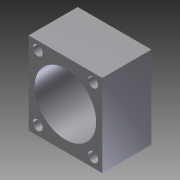
# Autodesk Inventor part: glass socket
Saved by Autodesk Inventor 2011 (Build 150239000, 239)
## iProperties
Created: 2013-10-30
Part Number: glass socket
Document SubType Name: Modeling
Designer: Devon
Density: 1 g/cm^3
Author: Devon
Autodesk Inventor part; units mm, degrees
ref_plane "YZ Plane" through (0, 0, 0) normal (1, 0, 0) x (0, 1, 0)
ref_plane "XZ Plane" through (0, 0, 0) normal (0, 1, 0) x (-1, 0, 0)
ref_plane "XY Plane" through (0, 0, 0) normal (0, 0, 1) x (1, 0, 0)
sketch "Sketch1" plane through (0, 0, 0) normal (0, 0, 1) x (1, 0, 0)
  line L0 (-26.7465, 47.6774) -> (49.4535, 47.6774)
  line L1 (49.4535, 47.6774) -> (49.4535, -37.4126)
  line L2 (49.4535, -37.4126) -> (-26.7465, -37.4126)
  line L3 (-26.7465, -37.4126) -> (-26.7465, 47.6774)
  line L4 (-26.7465, 47.6774) -> (-9.2459, 47.6774)
  line L5 (49.4535, 47.6774) -> (31.9529, 47.6774)
  line L6 (49.4535, 47.6774) -> (49.4535, 41.683)
  line L7 (49.4535, -37.4126) -> (49.4535, -31.4182)
  circle A0 centre (11.3535, 5.1324) radius 31.75
  line L8 (-26.7465, 47.6774) -> (-17.2215, 47.6774)
  line L9 (49.4535, 47.6774) -> (39.9285, 47.6774)
  line L10 (-26.7465, -37.4126) -> (-26.7465, -27.8876)
  circle A1 centre (-17.2215, -27.8876) radius 2.7813
  circle A2 centre (39.9285, -27.8876) radius 2.7813
  circle A3 centre (39.9285, 38.9906) radius 2.7813
  line L11 (-26.7465, -27.8876) -> (-17.2215, -27.8876)
  circle A4 centre (-17.2215, 38.9906) radius 2.7813
  point P0 (0, 0)
  dimension "d0" = 76.2
  dimension "d1" = 85.09
  dimension "d2" = 17.5006
  dimension "d3" = 17.5006
  dimension "d4" = 5.9944
  dimension "d5" = 5.9944
  dimension "d25" = 63.5
  dimension "d26" = 9.525
  dimension "d30" = 9.525
  dimension "d31" = 5.5626
  dimension "d32" = 5.5626
  dimension "d45" = 5.5626
  dimension "d46" = 9.525
  dimension "d48" = 5.5626
  constraints: 24 end point, 7 point on line, 5 centre point, 2 parallel, 1 coincident, 1 horizontal, 1 perpendicular
  measures "d0" distance of L1.end L2.end
  measures "d1" distance of L0.end L1.end
  measures "d2" distance of L0.start L4.end
  measures "d3" distance of L0.end L5.end
  measures "d4" distance of L0.end L6.end
  measures "d5" distance of L1.end L7.end
  measures "d25" diameter of A0
  measures "d26" distance of L0.start L8.end
  measures "d30" distance of L2.end L10.end
  measures "d31" diameter of A1
  measures "d32" diameter of A2
  measures "d45" diameter of A3
  measures "d46" distance of L10.end L11.end
  measures "d48" diameter of A4
extrude "Extrusion6" add sketch "Sketch1" along normal blind 12.7
sketch "Sketch4" plane through (0, 0, 12.7) normal (0, 0, 1) x (1, 0, 0)
  circle A0 centre (11.3535, 5.1324) radius 31.75 projected
  circle A1 centre (-17.2215, 38.9906) radius 2.7813 projected
  circle A2 centre (39.9285, -27.8876) radius 2.7813 projected
  circle A3 centre (-17.2215, -27.8876) radius 2.7813 projected
  circle A4 centre (39.9285, 38.9906) radius 2.7813 projected
  line L0 (-26.7465, 47.6774) -> (49.4535, 47.6774) projected
  line L1 (-26.7465, -37.4126) -> (-26.7465, 47.6774) projected
  line L2 (-26.7465, -37.4126) -> (49.4535, -37.4126)
  line L3 (49.4535, -37.4126) -> (49.4535, 47.6774)
  line L4 (49.4535, 47.6774) -> (-26.7465, 47.6774)
  line L5 (-26.7465, 47.6774) -> (-26.7465, -37.4126)
  circle A5 centre (11.3535, 5.1324) radius 31.75
  circle A6 centre (-17.2215, -27.8876) radius 5.1562
  circle A7 centre (-17.2215, 38.9906) radius 5.1562
  circle A8 centre (39.9285, 38.9906) radius 5.1562
  circle A9 centre (39.9285, -27.8876) radius 5.1562
  point P0 (0, 0)
  dimension "d51" = 10.3124
  dimension "d52" = 10.3124
  dimension "d53" = 10.3124
  dimension "d54" = 10.3124
  constraints: 8 end point, 5 centre point, 5 coincident, 2 parallel, 1 concentric, 1 horizontal, 1 perpendicular
  measures "d51" diameter of A6
  measures "d52" diameter of A7
  measures "d53" diameter of A8
  measures "d54" diameter of A9
extrude "Extrusion7" add sketch "Sketch4" along normal blind 38.1 contours L0 L3 L2 L1
body "Solid3"
